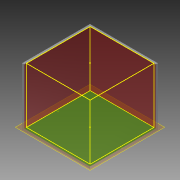
# Autodesk Inventor part: Box Pengukuran
Saved by Autodesk Inventor 2015 (Build 190159000, 159)
## iProperties
Created: 2015-02-05
Part Number: Box Pengukuran
Material: Generic
Document SubType Name: Modeling
Designer: Rafi Kurnia Putra
Density: 1 g/cm^3
Appearance: Clear
Mass: 2844 g
Surface Area: 5874 cm^2
Volume: 2844 cm^3
Author: Rafi Kurnia Putra
Autodesk Inventor part; units mm, degrees
ref_plane "YZ Plane" through (0, 0, 0) normal (1, 0, 0) x (0, 1, 0)
ref_plane "XY Plane" through (0, 0, 0) normal (0, 0, 1) x (1, 0, 0)
sketch "Sketch1" plane through (0, 0, 0) normal (0, 1, 0) x (-1, 0, 0)
  line L0 (155, 155) -> (-155, 155)
  line L1 (-155, 155) -> (-155, -155)
  line L2 (-155, -155) -> (155, -155)
  line L3 (155, -155) -> (155, 155)
  line L4 (155, 155) -> (-155, -155) construction
  line L5 (-155, 155) -> (155, -155) construction
  line L6 (165, -165) -> (-165, -165)
  line L7 (-165, -165) -> (-165, 165)
  line L8 (-165, 165) -> (165, 165)
  line L9 (165, 165) -> (165, -165)
  point P0 (0, 0)
  dimension "d0" = 310
  dimension "d1" = 310
  constraints: 20 end point, 4 parallel, 2 midpoint, 2 perpendicular, 1 horizontal, 3 other
  measures "d0" distance of L2.end L1.end
  measures "d1" distance of L1.end L0.end
extrude "Extrusion1" add sketch "Sketch1" along normal blind 10 contours L3 L2 L1 L0 | L6 L7 L8 L9
extrude "Extrusion2" add sketch "Sketch1" along normal blind 280
sketch "Sketch4" plane through (0, 280, 0) normal (0, 1, 0) x (1, 0, 0)
  line L0 (-155, 155) -> (-155, -155) projected
  line L1 (-155, -155) -> (155, -155) projected
  line L2 (155, -155) -> (155, 155) projected
  line L3 (155, 155) -> (-155, 155) projected
  point P0 (0, 0)
  dimension "d6" = 310
  dimension "d7" = 310
  measures "d6" distance of L1.end L2.end
  measures "d7" distance of L2.end L0.start
sketch "Sketch5" plane through (155, 10, 155) normal (-1, 0, 0) x (0, 0, 1)
  line L0 (0, 0) -> (-310, 0) projected
  line L1 (0, 0) -> (0, 270) projected
  line L2 (-310, 270) -> (0, 270) projected
  line L3 (-310, 0) -> (-310, 270) projected
  point P0 (-155, -10)
  dimension "d8" = 270
  measures "d8" distance between parallel lines of L0 L2
sketch "Sketch6" plane through (0, 10, 0) normal (0, 1, 0) x (1, 0, 0)
  line L0 (-155, 155) -> (-155, -155) projected
  line L1 (-155, -155) -> (155, -155) projected
  line L2 (155, -155) -> (155, 155) projected
  line L3 (155, 155) -> (-155, 155) projected
  point P0 (0, 0)
sketch "Sketch7" plane through (-155, 10, -155) normal (1, 0, 0) x (0, 0, -1)
  line L0 (0, 0) -> (-310, 0) projected
  line L1 (0, 0) -> (0, 270) projected
  line L2 (-310, 270) -> (0, 270) projected
  line L3 (-310, 0) -> (-310, 270) projected
  point P0 (-155, -10)
sketch "Sketch8" plane through (0, 280, 0) normal (0, 1, 0) x (1, 0, 0)
  line L0 (165, 165) -> (-165, 165)
  line L1 (155, 155) -> (155, 165)
  line L2 (-165, 165) -> (165, 165)
  line L3 (-155, 155) -> (-155, 165)
  line L4 (155, 155) -> (-155, 155)
  point P0 (0, 0)
  dimension "d0" = 310
  constraints: 10 end point, 2 point on line, 1 parallel, 1 perpendicular, 1 vertical
extrude "Extrusion3" cut sketch "Sketch8" against normal blind 270
sketch "Sketch9" plane through (0, 280, 0) normal (0, 1, 0) x (1, 0, 0)
  line L0 (-155, -155) -> (-155, 165) projected
  line L1 (-155, 165) -> (-165, 165) projected
  line L2 (-165, 165) -> (-165, -165) projected
  line L3 (-165, -165) -> (165, -165) projected
  line L4 (165, -165) -> (165, 165) projected
  line L5 (165, 165) -> (155, 165) projected
  line L6 (155, 165) -> (155, -155) projected
  line L7 (155, -155) -> (-155, -155) projected
  line L8 (-155, -155) -> (-165, -155)
  point P0 (0, 0)
  constraints: 2 end point, 1 perpendicular, 1 point on line
extrude "Extrusion4" cut sketch "Sketch9" against normal blind 270 contours L8 L2 L1 L0
ref_plane "Work Plane1" through (0, 10, 0) normal (0, 1, 0) x (-1, 0, 0)
body "Solid1"
